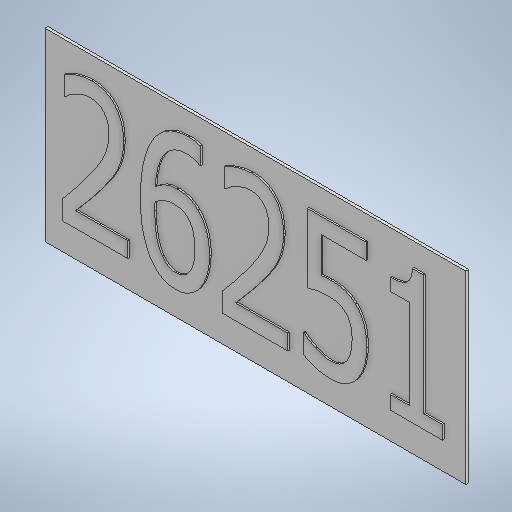
# Autodesk Inventor part: Alliance_Plate_V2
Saved by Autodesk Inventor 2025.1 (Build 291241000, 241)
## iProperties
Created: 2024-11-18
Part Number: Alliance_Plate_V2
Material: Generic
Document SubType Name: Modeling
Designer: ishaa
Density: 1 g/cm^3
Appearance: Default
Author: ishaa
Autodesk Inventor part; units mm, degrees
ref_plane "YZ Plane" through (0, 0, 0) normal (1, 0, 0) x (0, 1, 0)
ref_plane "XZ Plane" through (0, 0, 0) normal (0, 1, 0) x (-1, 0, 0)
ref_plane "XY Plane" through (0, 0, 0) normal (0, 0, 1) x (1, 0, 0)
sketch "Sketch1" plane through (0, 0, 0) normal (0, 0, 1) x (1, 0, 0)
  line L0 (-86.5, -38) -> (86.5, -38)
  line L1 (86.5, -38) -> (86.5, 38)
  line L2 (86.5, 38) -> (-86.5, 38)
  line L3 (-86.5, 38) -> (-86.5, -38)
  line L4 (-86.5, -38) -> (86.5, 38) construction
  line L5 (86.5, -38) -> (-86.5, 38) construction
  point P0 (0, 0)
  dimension "d0" = 173
  dimension "d1" = 76
  constraints: 12 end point, 2 midpoint, 2 parallel, 1 horizontal, 1 perpendicular
  measures "d0" distance of L2.end L1.end
  measures "d1" distance of L1.end L0.end
extrude "Extrusion1" add sketch "Sketch1" along normal blind 1.2
sketch "Sketch2" plane through (0, 0, 1.2) normal (0, 0, 1) x (1, 0, 0)
  line L0 (-81.9719, 29.6076) -> (2850.8468, 29.6076) construction
  line L1 (2850.8468, 29.6076) -> (2850.8468, -1197.0576) construction
  line L2 (2850.8468, -1197.0576) -> (-81.9719, -1197.0576) construction
  line L3 (-81.9719, -1197.0576) -> (-81.9719, 29.6076) construction
  line L4 (-51.7408, -26.3265) -> (-78.7756, -26.3265)
  line L5 (-78.7756, -26.3265) -> (-78.7756, -18.5579)
  spline S0 degree 2 poles (-78.7756, -18.5579) (-75.8457, -15.1397) (-70.6962, -8.7916) (-68.2103, -5.3734) knots 0 0 0 1 2 2 2
  spline S1 degree 2 poles (-68.2103, -5.3734) (-63.194, 1.5074) (-59.5538, 9.7644) (-59.5538, 14.1592) knots 0 0 0 1 2 2 2
  spline S2 degree 2 poles (-59.5538, 14.1592) (-59.5538, 16.4676) (-60.708, 19.9302) (-61.6846, 21.04) knots 0 0 0 1 2 2 2
  spline S3 degree 2 poles (-61.6846, 21.04) (-62.75, 22.1498) (-65.4136, 23.2596) (-67.0561, 23.2596) knots 0 0 0 1 2 2 2
  spline S4 degree 2 poles (-67.0561, 23.2596) (-68.6098, 23.2596) (-71.806, 22.2829) (-73.271, 21.5283) knots 0 0 0 1 2 2 2
  spline S5 degree 2 poles (-73.271, 21.5283) (-74.514, 20.9068) (-76.8224, 19.1311) (-77.5326, 18.5096) knots 0 0 0 1 2 2 2
  line L6 (-77.5326, 18.5096) -> (-77.8434, 18.5096)
  line L7 (-77.8434, 18.5096) -> (-77.8434, 26.3226)
  spline S6 degree 2 poles (-77.8434, 26.3226) (-76.0233, 27.4324) (-69.542, 29.6077) (-66.6122, 29.6077) knots 0 0 0 1 2 2 2
  spline S7 degree 2 poles (-66.6122, 29.6077) (-60.486, 29.6077) (-53.5609, 21.4839) (-53.5609, 14.5587) knots 0 0 0 1 2 2 2
  spline S8 degree 2 poles (-53.5609, 14.5587) (-53.5609, 11.3181) (-54.7595, 5.9022) (-55.8249, 3.5938) knots 0 0 0 1 2 2 2
  spline S9 degree 2 poles (-55.8249, 3.5938) (-56.9347, 1.1967) (-59.9533, -3.5089) (-61.6846, -5.7729) knots 0 0 0 1 2 2 2
  spline S10 degree 2 poles (-61.6846, -5.7729) (-64.4369, -9.5462) (-71.2289, -17.6256) (-73.271, -19.9784) knots 0 0 0 1 2 2 2
  line L8 (-73.271, -19.9784) -> (-51.7408, -19.9784)
  line L9 (-51.7408, -19.9784) -> (-51.7408, -26.3265)
  spline S11 degree 2 poles (-18.1803, -8.5696) (-18.1803, -12.7869) (-20.3999, -19.934) (-22.3088, -22.3312) knots 0 0 0 1 2 2 2
  spline S12 degree 2 poles (-22.3088, -22.3312) (-24.262, -24.8615) (-29.1452, -27.4807) (-32.0751, -27.4807) knots 0 0 0 1 2 2 2
  spline S13 degree 2 poles (-32.0751, -27.4807) (-35.0493, -27.4807) (-39.9325, -24.9947) (-41.7525, -22.5088) knots 0 0 0 1 2 2 2
  spline S14 degree 2 poles (-41.7525, -22.5088) (-44.0165, -19.5345) (-46.5913, -9.5462) (-46.5913, -2.2659) knots 0 0 0 1 2 2 2
  spline S15 degree 2 poles (-46.5913, -2.2659) (-46.5913, 4.8812) (-44.2385, 16.3788) (-41.7969, 20.6404) knots 0 0 0 1 2 2 2
  spline S16 degree 2 poles (-41.7969, 20.6404) (-39.3998, 24.8133) (-31.8531, 29.4745) (-26.9256, 29.4745) knots 0 0 0 1 2 2 2
  spline S17 degree 2 poles (-26.9256, 29.4745) (-25.4606, 29.4745) (-22.9303, 29.1193) (-21.9536, 28.7198) knots 0 0 0 1 2 2 2
  line L10 (-21.9536, 28.7198) -> (-21.9536, 21.6615)
  line L11 (-21.9536, 21.6615) -> (-22.22, 21.6615)
  spline S18 degree 2 poles (-22.22, 21.6615) (-23.019, 22.1942) (-26.0377, 23.1264) (-27.7246, 23.1264) knots 0 0 0 1 2 2 2
  spline S19 degree 2 poles (-27.7246, 23.1264) (-33.1849, 23.1264) (-39.9325, 13.8928) (-40.554, 4.8368) knots 0 0 0 1 2 2 2
  spline S20 degree 2 poles (-40.554, 4.8368) (-38.4675, 6.6569) (-34.0727, 8.6545) (-31.4536, 8.6545) knots 0 0 0 1 2 2 2
  spline S21 degree 2 poles (-31.4536, 8.6545) (-28.8788, 8.6545) (-25.0167, 7.3672) (-22.9303, 5.4139) knots 0 0 0 1 2 2 2
  spline S22 degree 2 poles (-22.9303, 5.4139) (-20.5331, 3.1499) (-18.1803, -3.864) (-18.1803, -8.5696) knots 0 0 0 1 2 2 2
  spline S23 degree 2 poles (-24.1732, -8.8804) (-24.1732, -5.5066) (-25.5938, -0.9342) (-27.1919, 0.664) knots 0 0 0 1 2 2 2
  spline S24 degree 2 poles (-27.1919, 0.664) (-28.3017, 1.8182) (-31.2316, 2.5728) (-32.7409, 2.5728) knots 0 0 0 1 2 2 2
  spline S25 degree 2 poles (-32.7409, 2.5728) (-34.8274, 2.5728) (-38.6895, 1.0191) (-40.554, -0.4459) knots 0 0 0 1 2 2 2
  spline S26 degree 2 poles (-40.554, -0.4459) (-40.6427, -1.2449) (-40.6871, -2.7542) (-40.6871, -3.9084) knots 0 0 0 1 2 2 2
  spline S27 degree 2 poles (-40.6871, -3.9084) (-40.6871, -9.5906) (-38.9114, -16.5602) (-37.5797, -18.3803) knots 0 0 0 1 2 2 2
  spline S28 degree 2 poles (-37.5797, -18.3803) (-36.2923, -20.1116) (-33.6288, -21.4877) (-32.0751, -21.4877) knots 0 0 0 1 2 2 2
  spline S29 degree 2 poles (-32.0751, -21.4877) (-28.5681, -21.4877) (-24.1732, -15.1841) (-24.1732, -8.8804) knots 0 0 0 1 2 2 2
  line L12 (14.0484, -26.3265) -> (-12.9864, -26.3265)
  line L13 (-12.9864, -26.3265) -> (-12.9864, -18.5579)
  spline S30 degree 2 poles (-12.9864, -18.5579) (-10.0565, -15.1397) (-4.907, -8.7916) (-2.4211, -5.3734) knots 0 0 0 1 2 2 2
  spline S31 degree 2 poles (-2.4211, -5.3734) (2.5952, 1.5074) (6.2354, 9.7644) (6.2354, 14.1592) knots 0 0 0 1 2 2 2
  spline S32 degree 2 poles (6.2354, 14.1592) (6.2354, 16.4676) (5.0812, 19.9302) (4.1046, 21.04) knots 0 0 0 1 2 2 2
  spline S33 degree 2 poles (4.1046, 21.04) (3.0392, 22.1498) (0.3756, 23.2596) (-1.2669, 23.2596) knots 0 0 0 1 2 2 2
  spline S34 degree 2 poles (-1.2669, 23.2596) (-2.8206, 23.2596) (-6.0168, 22.2829) (-7.4818, 21.5283) knots 0 0 0 1 2 2 2
  spline S35 degree 2 poles (-7.4818, 21.5283) (-8.7248, 20.9068) (-11.0332, 19.1311) (-11.7434, 18.5096) knots 0 0 0 1 2 2 2
  line L14 (-11.7434, 18.5096) -> (-12.0542, 18.5096)
  line L15 (-12.0542, 18.5096) -> (-12.0542, 26.3226)
  spline S36 degree 2 poles (-12.0542, 26.3226) (-10.2341, 27.4324) (-3.7528, 29.6077) (-0.823, 29.6077) knots 0 0 0 1 2 2 2
  spline S37 degree 2 poles (-0.823, 29.6077) (5.3032, 29.6077) (12.2283, 21.4839) (12.2283, 14.5587) knots 0 0 0 1 2 2 2
  spline S38 degree 2 poles (12.2283, 14.5587) (12.2283, 11.3181) (11.0298, 5.9022) (9.9643, 3.5938) knots 0 0 0 1 2 2 2
  spline S39 degree 2 poles (9.9643, 3.5938) (8.8545, 1.1967) (5.8359, -3.5089) (4.1046, -5.7729) knots 0 0 0 1 2 2 2
  spline S40 degree 2 poles (4.1046, -5.7729) (1.3523, -9.5462) (-5.4397, -17.6256) (-7.4818, -19.9784) knots 0 0 0 1 2 2 2
  line L16 (-7.4818, -19.9784) -> (14.0484, -19.9784)
  line L17 (14.0484, -19.9784) -> (14.0484, -26.3265)
  spline S41 degree 2 poles (46.4547, -8.9248) (46.4547, -12.8757) (44.4127, -19.6233) (42.5926, -22.1092) knots 0 0 0 1 2 2 2
  spline S42 degree 2 poles (42.5926, -22.1092) (40.7281, -24.5952) (35.2235, -27.4807) (31.8497, -27.4807) knots 0 0 0 1 2 2 2
  spline S43 degree 2 poles (31.8497, -27.4807) (28.6978, -27.4807) (22.5717, -25.7494) (20.3521, -24.3732) knots 0 0 0 1 2 2 2
  line L18 (20.3521, -24.3732) -> (20.3521, -16.6046)
  line L19 (20.3521, -16.6046) -> (20.7516, -16.6046)
  spline S44 degree 2 poles (20.7516, -16.6046) (21.4619, -17.2261) (23.9479, -18.8242) (25.5016, -19.5345) knots 0 0 0 1 2 2 2
  spline S45 degree 2 poles (25.5016, -19.5345) (27.2329, -20.2892) (30.1184, -21.1326) (31.8941, -21.1326) knots 0 0 0 1 2 2 2
  spline S46 degree 2 poles (31.8941, -21.1326) (33.6698, -21.1326) (37.0436, -19.5345) (38.2422, -17.8032) knots 0 0 0 1 2 2 2
  spline S47 degree 2 poles (38.2422, -17.8032) (39.3076, -16.1607) (40.4618, -11.8102) (40.4618, -8.8804) knots 0 0 0 1 2 2 2
  spline S48 degree 2 poles (40.4618, -8.8804) (40.4618, -5.9505) (39.2188, -2.2215) (37.9758, -0.9786) knots 0 0 0 1 2 2 2
  spline S49 degree 2 poles (37.9758, -0.9786) (36.7328, 0.3976) (33.0483, 1.5518) (30.7843, 1.5518) knots 0 0 0 1 2 2 2
  spline S50 degree 2 poles (30.7843, 1.5518) (28.3871, 1.5518) (23.5483, 0.6196) (22.1278, 0.22) knots 0 0 0 1 2 2 2
  line L20 (22.1278, 0.22) -> (22.1278, 28.4535)
  line L21 (22.1278, 28.4535) -> (46.1884, 28.4535)
  line L22 (46.1884, 28.4535) -> (46.1884, 22.0166)
  line L23 (46.1884, 22.0166) -> (27.7656, 22.0166)
  line L24 (27.7656, 22.0166) -> (27.7656, 7.4116)
  spline S51 degree 2 poles (27.7656, 7.4116) (28.831, 7.5891) (30.9174, 7.7223) (31.7609, 7.7223) knots 0 0 0 1 2 2 2
  spline S52 degree 2 poles (31.7609, 7.7223) (35.1347, 7.7223) (39.7959, 6.3462) (41.9267, 4.3041) knots 0 0 0 1 2 2 2
  spline S53 degree 2 poles (41.9267, 4.3041) (44.1019, 2.2621) (46.4547, -3.9528) (46.4547, -8.9248) knots 0 0 0 1 2 2 2
  line L25 (77.618, -26.3265) -> (56.2654, -26.3265)
  line L26 (56.2654, -26.3265) -> (56.2654, -20.7331)
  line L27 (56.2654, -20.7331) -> (64.2116, -20.7331)
  line L28 (64.2116, -20.7331) -> (64.2116, 15.9793)
  line L29 (64.2116, 15.9793) -> (56.2654, 15.9793)
  line L30 (56.2654, 15.9793) -> (56.2654, 20.9956)
  spline S54 degree 2 poles (56.2654, 20.9956) (60.749, 20.9956) (65.055, 24.1918) (65.277, 28.631) knots 0 0 0 1 2 2 2
  line L31 (65.277, 28.631) -> (69.8494, 28.631)
  line L32 (69.8494, 28.631) -> (69.8494, -20.7331)
  line L33 (69.8494, -20.7331) -> (77.618, -20.7331)
  line L34 (77.618, -20.7331) -> (77.618, -26.3265)
  point P0 (0, 0)
  constraints: 2 other
emboss "Emboss1" sketch "Sketch2" operation add depth 0.7 direction (0, 0, -1)
body "Solid1"
